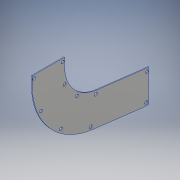
# Autodesk Inventor part: Storage Side Plate
Saved by Autodesk Inventor 2019.4 (Build 234330000, 330)
## iProperties
Created: 2020-01-11
Part Number: Storage Side Plate
Material: Aluminum 6061
Document SubType Name: Modeling
Designer: admin
Density: 2.7 g/cm^3
Appearance: Aluminum - Flat
Mass: 2247.91 g
Surface Area: 3432.51 cm^2
Volume: 832.56 cm^3
Author: admin
Autodesk Inventor part; units mm, degrees
ref_plane "YZ Plane" through (0, 0, 0) normal (1, 0, 0) x (0, 1, 0)
ref_plane "XZ Plane" through (0, 0, 0) normal (0, 1, 0) x (-1, 0, 0)
ref_plane "XY Plane" through (0, 0, 0) normal (0, 0, 1) x (1, 0, 0)
sketch "Sketch1" plane through (0, 0, 0) normal (1, 0, 0) x (0, 1, 0)
  arc A0 (-14.1738, -157.5454) -> (-242.5189, -360.0042) centre (-14.1738, -387.5454) ccw
  arc A1 (-14.1738, 45.6546) -> (-444.2568, -335.6721) centre (-14.1738, -387.5454) ccw
  line L0 (-242.5189, -360.0042) -> (-278.7026, -660.0042)
  line L1 (-444.2568, -335.6721) -> (-480.4405, -635.6721)
  line L2 (-240.9738, -388.9494) -> (-240.9738, -448.9494) projected
  line L3 (-451.1738, -381.4494) -> (-451.1738, -301.4494) projected
  arc A2 (-278.7026, -660.0042) -> (-280.1416, -683.9531) centre (-80.1416, -683.9531) ccw
  arc A3 (-480.4405, -635.6721) -> (-483.3416, -683.9531) centre (-80.1416, -683.9531) ccw
  line L4 (-483.3416, -683.9531) -> (-280.1416, -683.9531)
  line L5 (-240.9738, -388.9494) -> (-272.528, -650.5664) construction
  line L6 (-451.1738, -381.4494) -> (-466.1978, -506.0144) construction
  line L7 (-14.1738, 45.6546) -> (35.8262, 45.6546)
  line L8 (35.8262, 45.6546) -> (35.8262, -157.5454)
  line L9 (35.8262, -157.5454) -> (-14.1738, -157.5454)
  dimension "d4" = 203.2
  dimension "d6" = 5
  dimension "d7" = 1.3856
  dimension "d8" = 230
  dimension "d9" = 300
  dimension "d10" = 200
  dimension "d35" = 50
  constraints: 16 end point, 8 point on circle, 5 tangent, 4 centre point, 4 parallel, 2 coincident, 2 horizontal, 2 perpendicular, 1 line through centre
  measures "d4" distance of L7.start L9.end
  measures "d6" distance between parallel lines of L5 L0
  measures "d7" distance between parallel lines of L1 L6
  measures "d8" radius of A0
  measures "d9" vertical distance of L0.start L0.end
  measures "d10" radius of A2
  measures "d35" distance of L7.start L7.end
extrude "Extrusion1" add sketch "Sketch1" along normal blind 5
sketch "Sketch2" plane through (5, 0, 0) normal (1, 0, 0) x (0, 0, -1)
  line L0 (672.5546, -300.3612) -> (352.375, -261.7436) construction
  line L1 (352.375, -261.7436) -> (234.9079, -212.1682) construction
  line L2 (234.9079, -212.1682) -> (157.1195, -111.1473) construction
  line L3 (157.1195, -111.1473) -> (145.5454, 15.8262) construction
  circle A0 centre (672.5546, -300.3612) radius 9.5
  circle A1 centre (352.375, -261.7436) radius 9.5
  circle A2 centre (234.9079, -212.1682) radius 9.5
  circle A3 centre (157.1195, -111.1473) radius 9.5
  circle A4 centre (145.5454, 15.8262) radius 9.5
  line L4 (660.0042, -278.7026) -> (360.0042, -242.5189) construction
  circle A5 centre (72.4572, -74.3053) radius 88.9 construction
  line L5 (234.9079, -212.1682) -> (247.1189, -196.3286) construction
  arc A6 (157.5454, -14.1738) -> (360.0042, -242.5189) centre (387.5454, -14.1738) ccw construction
  line L6 (157.1195, -111.1473) -> (175.5536, -103.3895) construction
  line L7 (668.0222, -464.1974) -> (320.5405, -422.2868) construction
  line L8 (320.5405, -422.2868) -> (134.9837, -341.201) construction
  line L9 (134.9837, -341.201) -> (9.9307, -181.9276) construction
  line L10 (9.9307, -181.9276) -> (-33.6546, 15.8262) construction
  circle A7 centre (668.0222, -464.1974) radius 9.5
  circle A8 centre (320.5405, -422.2868) radius 9.5
  circle A9 centre (134.9837, -341.201) radius 9.5
  circle A10 centre (9.9307, -181.9276) radius 9.5
  circle A11 centre (-33.6546, 15.8262) radius 9.5
  line L11 (-33.6546, 15.8262) -> (145.5454, 15.8262) construction
  line L12 (335.6721, -444.2568) -> (635.6721, -480.4405) projected
  circle A12 centre (145.5454, 15.8262) radius 25.4 construction
  circle A13 centre (-33.6546, 15.8262) radius 25.4 construction
  line L13 (9.9307, -181.9276) -> (-8.3469, -190.0473) construction
  arc A14 (-45.6546, -14.1738) -> (335.6721, -444.2568) centre (387.5454, -14.1738) ccw projected
  line L14 (157.5454, 35.8262) -> (-45.6546, 35.8262) projected
  line L15 (683.9531, -483.3416) -> (683.9531, -280.1416) projected
  line L16 (134.9837, -341.201) -> (122.759, -357.03) construction
  point P0 (0, 0)
  dimension "d11" = 322.5
  dimension "d12" = 19
  dimension "d13" = 19
  dimension "d14" = 19
  dimension "d15" = 19
  dimension "d16" = 19
  dimension "d18" = 12
  dimension "d19" = 20
  dimension "d20" = 177.8
  dimension "d21" = 20
  dimension "d22" = 20
  dimension "d23" = 19
  dimension "d24" = 19
  dimension "d25" = 19
  dimension "d26" = 19
  dimension "d28" = 19
  dimension "d29" = 20
  dimension "d30" = 50.8
  dimension "d31" = 50.8
  dimension "d34" = 20
  dimension "d36" = 20
  dimension "d37" = 15.9309
  dimension "d38" = 20
  dimension "d39" = 202.5
  dimension "d40" = 127.5
  dimension "d41" = 350
  dimension "d42" = 202.5
  dimension "d43" = 202.5
  dimension "d44" = 127.5
  dimension "d46" = 127.5
  dimension "d49" = 12
  constraints: 26 end point, 13 centre point, 11 coincident, 4 line through centre, 4 point on circle, 1 horizontal, 1 parallel
  measures "d11" distance of L0.start L0.end
  measures "d12" diameter of A0
  measures "d13" diameter of A1
  measures "d14" diameter of A2
  measures "d15" diameter of A3
  measures "d16" diameter of A4
  measures "d18" horizontal distance of A6.start L11.end
  measures "d19" distance from line of L4 A1.centre
  measures "d20" diameter of A5
  measures "d21" distance of L5.start L5.end
  measures "d22" distance of L6.start L6.end
  measures "d23" diameter of A7
  measures "d24" diameter of A8
  measures "d25" diameter of A9
  measures "d26" diameter of A10
  measures "d28" diameter of A11
  measures "d29" distance between parallel lines of L12 L7
  measures "d30" diameter of A12
  measures "d31" diameter of A13
  measures "d34" distance of L13.start L13.end
  measures "d36" distance from line of L14 L11.end
  measures "d37" distance from line of L15 L7.start
  measures "d38" distance of L16.start L16.end
  measures "d39" distance of L7.end L8.end
  measures "d40" distance of L0.end L1.end
  measures "d41" distance of L7.start L7.end
  measures "d42" distance of L8.end L9.end
  measures "d43" distance of L10.end L9.end
  measures "d44" distance of L1.end L2.end
  measures "d46" distance of L2.end L3.end
  measures "d49" horizontal distance of L14.end L10.end
extrude "Extrusion2" cut sketch "Sketch2" against normal through all
body "Solid1"
